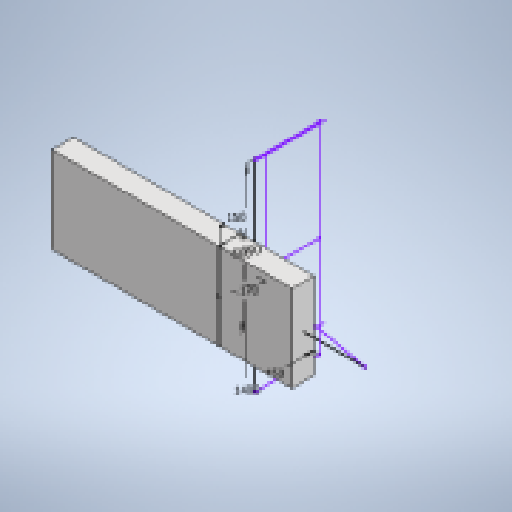
# Autodesk Inventor part: MSC DIM 012 carriage nose
Saved by Autodesk Inventor 2025.1 (Build 291241020, 241B)
## iProperties
Created: 2024-11-21
Part Number: MSC DIM 012 carriage nose
Material: Generic
Document SubType Name: Modeling
Designer: user
Density: 1 g/cm^3
Appearance: Default
Author: user
Autodesk Inventor part; units mm, degrees
ref_plane "YZ Plane" through (0, 0, 0) normal (1, 0, 0) x (0, 1, 0)
ref_plane "XZ Plane" through (0, 0, 0) normal (0, 1, 0) x (-1, 0, 0)
ref_plane "XY Plane" through (0, 0, 0) normal (0, 0, 1) x (1, 0, 0)
sketch "Sketch1" plane through (0, 0, 0) normal (1, 0, 0) x (0, 1, 0)
  line L0 (0, -300) -> (150, -300)
  line L1 (150, -300) -> (150, 300)
  line L2 (150, 300) -> (0, 300)
  line L3 (0, 300) -> (0, -300)
  line L4 (150, -110.5085) -> (250, -110.5085)
  line L5 (250, -110.5085) -> (250, 120.1522)
  line L6 (250, 120.1522) -> (150, 120.1522)
  line L7 (150, 120.1522) -> (150, -110.5085)
  line L8 (250, -527.4169) -> (326.5108, -527.4169)
  line L9 (326.5108, -527.4169) -> (326.5108, 687.4915)
  line L10 (326.5108, 687.4915) -> (250, 687.4915)
  line L11 (250, 687.4915) -> (250, -527.4169)
  line L12 (326.5108, -527.4169) -> (729.0925, -527.4169)
  line L13 (326.5108, 687.4915) -> (739.1213, 687.4915)
  point P0 (0, 0)
  point P1 (0, 0)
  dimension "d0" = 600
  dimension "d1" = 150
  dimension "d2" = 100
  constraints: 28 end point, 6 parallel, 5 horizontal, 3 perpendicular, 2 point on line, 1 coincident, 1 midpoint
  measures "d0" distance between parallel lines of L2 L0
  measures "d1" distance of L1.end L2.end
  measures "d2" distance of L5.end L6.end
sketch "Sketch2" plane through (0, 0, 0) normal (1, 0, 0) x (0, 1, 0)
  line L0 (0, -300) -> (150, -300)
  line L1 (150, -300) -> (150, 300)
  line L2 (150, 300) -> (0, 300)
  line L3 (0, 300) -> (0, -300)
  point P0 (0, 0)
  point P1 (0, 0)
  dimension "d3" = 600
  dimension "d4" = 150
  constraints: 8 end point, 2 parallel, 1 coincident, 1 horizontal, 1 midpoint, 1 perpendicular
  measures "d3" distance of L0.end L1.end
  measures "d4" distance of L1.end L2.end
extrude "Extrusion1" add sketch "Sketch2" along normal blind 507.75 and the other way blind 1159.5
sketch "Sketch3" plane through (-1159.5, 150, 300) normal (0, 1, 0) x (1, 0, 0)
  circle A0 centre (1159.5, 300) radius 75
  dimension "d9" = 150
  constraints: 1 centre point, 1 coincident
  measures "d9" diameter of A0
extrude "Extrusion2" add sketch "Sketch3" along normal blind 100
sketch3d "3D Sketch1"
equation "\"d3\" = d0"
equation "\"d4\" = d1"
equation "\"d10\" = d2"
body "Solid1"
